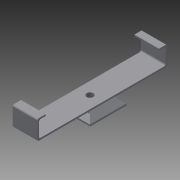
# Autodesk Inventor part: Tripod
Saved by Autodesk Inventor 2015 (Build 190159000, 159)
## iProperties
Created: 2015-08-12
Part Number: Tripod
Material: Generic
Document SubType Name: Modeling
Designer: Kurtis
Density: 1 g/cm^3
Appearance: Default
Author: Kurtis
Autodesk Inventor part; units mm, degrees
ref_plane "YZ Plane" through (0, 0, 0) normal (1, 0, 0) x (0, 1, 0)
ref_plane "XZ Plane" through (0, 0, 0) normal (0, 1, 0) x (-1, 0, 0)
ref_plane "XY Plane" through (0, 0, 0) normal (0, 0, 1) x (1, 0, 0)
sketch "Sketch1" plane through (0, 0, 0) normal (0, 0, 1) x (1, 0, 0)
  line L0 (0, 0) -> (43.5, 0)
  line L1 (43.5, 0) -> (43.5, 43.5)
  line L2 (43.5, 43.5) -> (0, 43.5)
  line L3 (0, 43.5) -> (0, 0)
  dimension "d0" = 43.5
  dimension "d1" = 43.5
  constraints: 8 end point, 2 parallel, 1 horizontal, 1 perpendicular
  measures "d0" distance of L2.end L1.end
  measures "d1" distance of L1.end L0.end
extrude "Extrusion1" add sketch "Sketch1" along normal blind 9
chamfer "Chamfer1" distance 7 angle 45 4 edges at (21.75, 43.5, 9) (0, 21.75, 9) (21.75, 0, 9) (43.5, 21.75, 9)
sketch "Sketch2" plane through (0, 0, 9) normal (0, 0, 1) x (1, 0, 0)
  line L0 (7, 7) -> (36.5, 7)
  line L1 (36.5, 7) -> (36.5, 36.5)
  line L2 (36.5, 36.5) -> (7, 36.5)
  line L3 (7, 36.5) -> (7, 7)
  point P0 (0, 0)
  constraints: 8 end point, 2 parallel, 1 horizontal, 1 perpendicular
extrude "Extrusion2" add sketch "Sketch2" along normal blind 2
sketch "Sketch3" plane through (36.5, 7, 9) normal (1, 0, 0) x (0, 0, -1)
  line L0 (0, 0) -> (0, 29.5) projected
  line L1 (-2, 90.75) -> (-2, -61.25)
  line L2 (-23.5, -63.25) -> (-23.5, -53.25)
  line L3 (-23.5, -53.25) -> (-21.5, -53.25)
  line L4 (-21.5, -53.25) -> (-21.5, -61.25)
  line L5 (-21.5, -61.25) -> (-2, -61.25)
  line L6 (-23.5, 92.75) -> (-23.5, 82.75)
  line L7 (-23.5, 82.75) -> (-21.5, 82.75)
  line L8 (-21.5, 82.75) -> (-21.5, 90.75)
  line L9 (-21.5, 90.75) -> (-2, 90.75)
  line L10 (-23.5, -63.25) -> (0, -63.25)
  line L11 (0, -63.25) -> (0, 92.75)
  line L12 (-23.5, 92.75) -> (0, 92.75)
  line L13 (9, -7) -> (9, 36.5) projected
  dimension "d15" = 10
  dimension "d16" = 2
  dimension "d17" = 8
  dimension "d21" = 156
  dimension "d22" = 23.5
  dimension "d23" = 19.5
  dimension "d24" = 2
  dimension "d27" = 9
  dimension "d28" = 63.25
  constraints: 24 end point, 6 perpendicular, 5 equal length, 1 horizontal, 1 parallel, 1 vertical
  measures "d15" distance of L2.start L2.end
  measures "d16" distance of L2.end L3.end
  measures "d17" distance of L3.end L4.end
  measures "d21" distance of L10.end L11.end
  measures "d22" distance of L2.start L10.end
  measures "d23" distance of L4.end L1.end
  measures "d24" distance between parallel lines of L10 L5
  measures "d27" distance between parallel lines of L11 L13
  measures "d28" distance of L10.end L0.start
extrude "Extrusion3" add sketch "Sketch3" against normal blind 29.5
fillet "Fillet1" radius 1 2 edges at (21.75, 36.5, 9) (21.75, 7, 9)
fillet "Fillet2" radius 2 8 edges at (21.75, -56.25, 9) (21.75, 99.75, 9) (21.75, 99.75, 32.5) (21.75, -56.25, 32.5) (21.75, -54.25, 30.5) (21.75, -54.25, 11) (21.75, 97.75, 11) (21.75, 97.75, 30.5)
sketch "Sketch4" plane through (0, 0, 0) normal (0, 0, -1) x (-1, 0, 0)
  line L0 (0, 0) -> (-43.5, 43.5) construction
  line L1 (-38.2071, 38.2071) -> (-43.5, 43.5) construction
  line L2 (-43.5, 43.5) -> (-43.5, 0) construction
  line L3 (-43.5, 0) -> (0, 43.5) construction
  circle A0 centre (-21.75, 21.75) radius 6.625
  dimension "d33" = 13.25
  constraints: 6 end point, 1 centre point, 1 collinear, 1 midpoint, 1 perpendicular, 1 vertical
  measures "d33" diameter of A0
extrude "Extrusion4" cut sketch "Sketch4" against normal blind 8
sketch "Sketch5" plane through (21.75, 21.75, 8) normal (0, 0, -1) x (-1, 0, 0)
  circle A0 centre (0, 0) radius 4
  point P0 (21.75, -21.75)
  dimension "d36" = 8
  constraints: 1 centre point
  measures "d36" diameter of A0
extrude "Extrusion5" cut sketch "Sketch5" against normal blind 44.75
body "Solid1"
